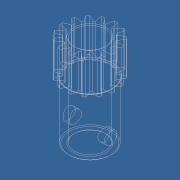
# Autodesk Inventor part: ENGR.RETA MOTORA(18)
Saved by Autodesk Inventor 2012 SP1 (Build 160190100, 190)
## iProperties
Created: 2012-07-24
Part Number: ENGR.RETA MOTORA(18)
Material: Carbon Steel
Document SubType Name: Modeling
Designer: bruno.silveira
Mass: 53.59 g
Surface Area: 20.5617 cm^2
Volume: 6.8094 cm^3
Density: 7.87 g/cm^3
Author: bruno.silveira
Autodesk Inventor part; units mm, degrees
ref_plane "YZ Plane" through (0, 0, 0) normal (1, 0, 0) x (0, 1, 0)
ref_plane "XZ Plane" through (0, 0, 0) normal (0, 1, 0) x (-1, 0, 0)
ref_plane "XY Plane" through (0, 0, 0) normal (0, 0, 1) x (1, 0, 0)
sketch "Sketch1" plane through (0, 0, 0) normal (0, 0, 1) x (1, 0, 0)
  circle A0 centre (0, 0) radius 8.5
  dimension "d0" = 17
  constraints: 1 centre point, 1 coincident
  measures "d0" diameter of A0
extrude "Extrusion1" add sketch "Sketch1" along normal blind 30
sketch "Sketch2" plane through (0, 0, 0) normal (0, 0, -1) x (-1, 0, 0)
  circle A0 centre (0, 0) radius 8.5 projected
  circle A1 centre (0, 0) radius 7
  dimension "d3" = 14
  constraints: 1 centre point, 1 coincident
  measures "d3" diameter of A1
extrude "Extrusion2" cut sketch "Sketch2" against normal blind 19
sketch "Sketch3" plane through (0, 0, 0) normal (0, 0, -1) x (-1, 0, 0)
  circle A0 centre (0, 0) radius 7 projected
  circle A1 centre (0, 0) radius 5
  dimension "d6" = 10
  constraints: 1 centre point, 1 coincident
  measures "d6" diameter of A1
extrude "Extrusion3" cut sketch "Sketch3" against normal blind 30 contours A1
chamfer "Chamfer1" distance 0.3 angle 45 3 edges at (5, 0, 0) (7, 0, 0) (5, 0, 30)
fillet "Fillet1" radius 0.3 1 edges at (7, 0, 19)
spur gear teeth "Spur Gear1" teeth 15 pitch diameter 15 tip diameter 16.9991 root diameter 12.5 face width 11 trims to tip circle yes start plane through (0, 0, 30) normal (0, 0, 1) x (1, 0, 0)
sketch "Sketch4" plane through (0, 0, 0) normal (1, 0, 0) x (0, 1, 0)
  circle A0 centre (0, 5) radius 2
  line L0 (6.7, 0) -> (-6.7, 0) projected
  point P0 (0, 0)
  dimension "d13" = 4
  dimension "d14" = 5
  constraints: 1 centre point
  measures "d13" diameter of A0
  measures "d14" distance from line of L0 A0.centre
extrude "Extrusion4" cut sketch "Sketch4" along normal mid plane 20
body "Solid1"
